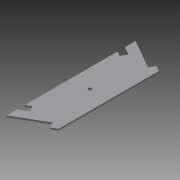
# Autodesk Inventor part: Triangle End
Saved by Autodesk Inventor 2015 (Build 190159000, 159)
## iProperties
Created: 2016-03-22
Part Number: Triangle End
Material: Generic
Document SubType Name: Modeling
Designer: Mac
Density: 1 g/cm^3
Appearance: Default
Author: Mac
Autodesk Inventor part; units mm, degrees
ref_plane "YZ Plane" through (0, 0, 0) normal (1, 0, 0) x (0, 1, 0)
ref_plane "XZ Plane" through (0, 0, 0) normal (0, 1, 0) x (-1, 0, 0)
ref_plane "XY Plane" through (0, 0, 0) normal (0, 0, 1) x (1, 0, 0)
sketch "Sketch1" plane through (0, 0, 0) normal (0, 1, 0) x (-1, 0, 0)
  line L0 (4.1559, 203.2) -> (4.1559, -203.2)
  line L1 (4.1559, -203.2) -> (156.5559, -291.1882)
  line L2 (4.1559, 203.2) -> (156.5559, 291.1882)
  line L3 (4.1559, 203.2) -> (180.1322, 203.2) construction
  line L4 (156.5559, 291.1882) -> (156.5559, -291.1882)
  point P0 (0, 0)
  point P1 (4.1559, 0)
  dimension "d0" = 120
  dimension "d1" = 30
  dimension "d2" = 406.4
  dimension "d5" = 152.4
  constraints: 10 end point, 2 vertical, 1 equal length, 1 horizontal, 1 horizontal alignment, 1 midpoint
  measures "d0" angle of L1 L0
  measures "d1" angle of L3 L2
  measures "d2" distance of L0.start L0.end
  measures "d5" distance between parallel lines of L0 L4
extrude "Extrusion1" add sketch "Sketch1" along normal blind 6.35
sketch "Sketch3" plane through (0, 6.35, 0) normal (0, 1, 0) x (1, 0, 0)
  line L0 (-1236.8748, 812.4936) -> (-137.0225, 177.4936) projected
  line L1 (-1224.1748, 834.4907) -> (-1236.8748, 812.4936) projected
  line L2 (-124.3225, 199.4907) -> (-1224.1748, 834.4907) projected
  line L3 (-137.0225, 177.4936) -> (-124.3225, 199.4907) projected
  line L4 (-26.6836, 216.2064) -> (-1258.5181, 927.4064) projected
  line L5 (-39.3836, 194.2093) -> (-26.6836, 216.2064) projected
  line L6 (-1271.2181, 905.4093) -> (-39.3836, 194.2093) projected
  line L7 (-1258.5181, 927.4064) -> (-1271.2181, 905.4093) projected
  line L8 (-1258.5181, -927.4064) -> (-26.6836, -216.2064) projected
  line L9 (-1271.2181, -905.4093) -> (-1258.5181, -927.4064) projected
  line L10 (-39.3836, -194.2093) -> (-1271.2181, -905.4093) projected
  line L11 (-26.6836, -216.2064) -> (-39.3836, -194.2093) projected
  line L12 (-137.0225, -177.4936) -> (-1236.8748, -812.4936) projected
  line L13 (-124.3225, -199.4907) -> (-137.0225, -177.4936) projected
  line L14 (-1224.1748, -834.4907) -> (-124.3225, -199.4907) projected
  line L15 (-1236.8748, -812.4936) -> (-1224.1748, -834.4907) projected
  line L16 (-156.5559, 291.1882) -> (-156.5559, -291.1882) projected
  line L17 (-156.5559, -218.1006) -> (-156.5559, -188.7712)
  line L18 (-156.5559, -188.7712) -> (-137.0225, -177.4936)
  line L19 (-137.0225, -177.4936) -> (-124.3225, -199.4907)
  line L20 (-124.3225, -199.4907) -> (-156.5559, -218.1006)
  line L21 (-136.8366, -176.7997) -> (-157.0639, -188.4779)
  line L22 (-157.0639, -188.4779) -> (-157.0639, -218.9805)
  line L23 (-157.0639, -218.9805) -> (-123.6286, -199.6766)
  line L24 (-123.6286, -199.6766) -> (-136.8366, -176.7997)
  line L25 (-156.5559, -261.8588) -> (-156.5559, -291.1882)
  line L26 (-156.5559, -291.1882) -> (-26.6836, -216.2064)
  line L27 (-156.5559, -291.1882) -> (-4.1559, -203.2) projected
  line L28 (-26.6836, -216.2064) -> (-39.3836, -194.2093)
  line L29 (-39.3836, -194.2093) -> (-156.5559, -261.8588)
  line L30 (-157.0639, -261.5655) -> (-157.0639, -292.0681)
  line L31 (-157.0639, -292.0681) -> (-25.9896, -216.3923)
  line L32 (-25.9896, -216.3923) -> (-39.1976, -193.5154)
  line L33 (-39.1976, -193.5154) -> (-157.0639, -261.5655)
  line L34 (-156.5559, 218.1006) -> (-156.5559, 188.7712)
  line L35 (-156.5559, 188.7712) -> (-137.0225, 177.4936)
  line L36 (-137.0225, 177.4936) -> (-124.3225, 199.4907)
  line L37 (-124.3225, 199.4907) -> (-156.5559, 218.1006)
  line L38 (-157.0639, 218.9805) -> (-157.0639, 188.4779)
  line L39 (-157.0639, 188.4779) -> (-136.8366, 176.7997)
  line L40 (-136.8366, 176.7997) -> (-123.6286, 199.6766)
  line L41 (-123.6286, 199.6766) -> (-157.0639, 218.9805)
  line L42 (-156.5559, 261.8588) -> (-156.5559, 291.1882)
  line L43 (-156.5559, 291.1882) -> (-26.6836, 216.2064)
  line L44 (-26.6836, 216.2064) -> (-39.3836, 194.2093)
  line L45 (-39.3836, 194.2093) -> (-156.5559, 261.8588)
  line L46 (-157.0639, 261.5655) -> (-157.0639, 292.0681)
  line L47 (-157.0639, 292.0681) -> (-25.9896, 216.3923)
  line L48 (-25.9896, 216.3923) -> (-39.1976, 193.5154)
  line L49 (-39.1976, 193.5154) -> (-157.0639, 261.5655)
  point P0 (0, 0)
  dimension "d6" = 0.508
  dimension "d7" = 0.508
  dimension "d8" = 0.508
  dimension "d9" = 0.508
  constraints: 64 end point, 12 point on line, 11 collinear, 4 perpendicular, 1 vertical, 12 other
  measures "d6" distance between parallel lines of L24 L13
  measures "d7" distance between parallel lines of L33 L29
  measures "d8" distance between parallel lines of L41 L37
  measures "d9" distance between parallel lines of L49 L6
extrude "Extrusion2" cut sketch "Sketch3" against normal through all contours L16 L2 L3 L0 | L16 L39 L38 L0 | L0 L38 L2 L16 | L0 L3 L2 L16 L41 L40 L39 | L49 L46 L6 L16 | L16 L6 L5 L4 L46 L47 L48 L49 | L33 L32 L27 L11 L10 L16 | L16 L10 L30 L33 | L21 L24 L23 L16 L14 L13 L12 | L16 L12 L22 L21 | L0 L1 L2 L38 | L2 L38 L41 L16 | L16 L14 L22 L12 | L12 L13 L14 L16 | L16 L4 L5 L6 | L6 L46 L4 L16 | L22 L14 L15 L12 | L16 L23 L22 L14 | L16 L8 L30 L10 | L10 L11 L8 L16 | L8 L27 L32 L31 L30
sketch "Sketch4" plane through (0, 6.35, 0) normal (0, 1, 0) x (1, 0, 0)
  line L0 (-4.1559, -203.2) -> (-4.1559, 203.2) projected
  point P0 (0, 0)
  point P1 (-80.3559, 0)
  dimension "d12" = 76.2
  dimension "d13" = 203.2
  measures "d12" distance from line of L0 point (-80.356, 0)
  measures "d13" vertical distance of L0.end point (-80.356, 0)
hole "Hole1" at (-80.3559, 6.35, 0) direction (0, -1, 0) diameter 13.4925 end through all
body "Solid1"
